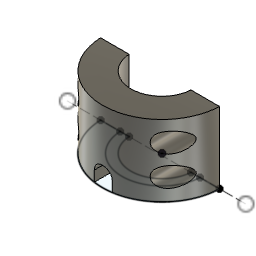
sphere_PS3 v1 (Autodesk Fusion 360 design; units mm, degrees)
Autodesk Fusion 360 part; units mm, degrees
sketch "Skizze1" plane through (0, 0, 0) normal (0, 0, 1) x (1, 0, 0)
  line L0 (-46.6781, -1) -> (43.3215, -1) construction
  arc A0 (-29.9833, -1) -> (29.9833, -1) centre (0, 0) ccw
  arc A1 (-20.1252, -1) -> (20.1252, -1) centre (0, 0) ccw
  arc A2 (-15.618, -1) -> (15.618, -1) centre (0, 0) ccw
  line L1 (15.618, -1) -> (29.9833, -1)
  line L2 (-15.618, -1) -> (-29.9833, -1)
  point P0 (-29.9833, -1)
  point P1 (-20.1252, -1)
  point P2 (-15.618, -1)
  point P3 (15.618, -1)
  point P4 (20.1252, -1)
  point P5 (29.9833, -1)
  dimension "d6" = 1
  dimension "d7" = 30
  dimension "d8" = 20.15
  dimension "d9" = 15.65
  constraint horizontal L0
  constraint coincident L0 P0
  constraint coincident L0 P1
  constraint coincident L0 P2
  constraint coincident L0 P3
  constraint coincident L0 P4
  constraint coincident L0 P5
  constraint coincident P5 A0.end
  constraint coincident P0 A0.start
  constraint coincident A0.centre A1.centre
  constraint coincident P4 A1.end
  constraint coincident P1 A1.start
  constraint coincident P3 A2.end
  constraint coincident P2 A2.start
  measures "d6" distance of A0.centre L0
  measures "d7" radius of A0
  measures "d8" radius of A1
  measures "d9" radius of A2
extrude "Extrusion1" add sketch "Skizze1" along normal blind 36
extrude "Extrusion2" cut sketch "Skizze1" along normal blind 5.3 contours A1 A2 L1 L2
sketch "Skizze3" plane through (0, -1, 0) normal (0, 1, 0) x (-1, 0, 0)
  line L0 (20.1252, 5.3) -> (20.1252, 0)
  line L1 (20.1252, 0) -> (29.9833, 0)
  line L2 (29.9833, 0) -> (29.9833, 36)
  line L3 (29.9833, 36) -> (15.618, 36)
  line L4 (15.618, 36) -> (15.618, 5.3)
  line L5 (15.618, 5.3) -> (20.1252, 5.3)
  line L6 (-23, 38.9334) -> (-23, -25) construction
  line L7 (23, 38.9334) -> (23, -33.2487) construction
  line L8 (-52.1355, 10.8) -> (51.6739, 10.8) construction
  line L9 (-50.0712, 25.8) -> (44.4743, 25.8) construction
  circle A0 centre (-23, 25.8) radius 1.75
  circle A1 centre (-23, 10.8) radius 1.75
  circle A2 centre (23, 25.8) radius 1.75
  circle A3 centre (23, 10.8) radius 1.75
  line L10 (-51.02, 5.3) -> (55, 5.3) construction
  line L11 (0, 38.1175) -> (0, -20) construction
  line L12 (-4.5, 5.3) -> (4.5, 5.3)
  line L13 (4.5, 5.3) -> (4.5, -4.7)
  line L14 (4.5, -4.7) -> (-4.5, -4.7)
  line L15 (-4.5, -4.7) -> (-4.5, 5.3)
  arc A4 (4.5, 5.3) -> (-4.5, 5.3) centre (0, 5.3) ccw
  point P0 (-23, 25.8)
  point P1 (-23, 10.8)
  point P2 (23, 25.8)
  point P3 (23, 10.8)
  dimension "d14" = 10.8
  dimension "d15" = 25.8
  dimension "d17" = 3.5
  dimension "d18" = 3.5
  dimension "d19" = 3.5
  dimension "d20" = 3.5
  dimension "d21" = 5.3
  dimension "d29" = 23
  dimension "d30" = 23
  constraint vertical L6
  constraint perpendicular L3 L7
  constraint horizontal L8
  constraint perpendicular L2 L9
  constraint coincident L9 P0
  constraint coincident L6 P0
  constraint coincident L6 P1
  constraint coincident L8 P1
  constraint coincident L9 P2
  constraint coincident L7 P2
  constraint coincident L7 P3
  constraint coincident L8 P3
  constraint coincident P0 A0.centre
  constraint coincident P1 A1.centre
  constraint coincident P2 A2.centre
  constraint coincident P3 A3.centre
  constraint horizontal L10
  constraint vertical L11
  constraint coincident origin L11
  constraint horizontal L12
  constraint vertical L13
  constraint horizontal L14
  constraint vertical L15
  constraint midpoint L12 A4.centre
  measures "d14" distance of L8 origin
  measures "d15" distance of origin L9
  measures "d17" diameter of A3
  measures "d18" diameter of A2
  measures "d19" diameter of A0
  measures "d20" diameter of A1
  measures "d21" distance of origin L10
  measures "d29" distance of L6 L11
  measures "d30" distance of L7 L11
extrude "Extrusion3" cut sketch "Skizze3" against normal blind 100 contours A0 | A1 | A2 | A3 | L12 A4 | L12 L13 L14 L15
ref_plane "Arbeitsebene1" through (0, -30, 0) normal (0, 1, 0) x (0, 0, 1)
sketch "Skizze5" plane through (0, -30, 0) normal (0, 1, 0) x (1, 0, 0)
  line L0 (23, -32.4719) -> (23, 19) construction
  line L1 (-23, -30.4738) -> (-23, 19) construction
  line L2 (48, -10.8) -> (-39, -10.8) construction
  line L3 (47, -25.8) -> (-45, -25.8) construction
  circle A0 centre (23, -25.8) radius 5
  circle A1 centre (23, -10.8) radius 5
  circle A2 centre (-23, -25.8) radius 5
  circle A3 centre (-23, -10.8) radius 5
  dimension "d27" = 23
  dimension "d31" = 23
  dimension "d32" = 10.8
  dimension "d33" = 25.8
  dimension "d34" = 10
  dimension "d35" = 10
  dimension "d36" = 10
  dimension "d37" = 10
  constraint vertical L0
  constraint vertical L1
  constraint perpendicular L1 L2
  constraint perpendicular L0 L3
  constraint coincident L0 A0.centre
  constraint coincident L3 A0.centre
  constraint coincident L2 A1.centre
  constraint coincident L0 A1.centre
  constraint coincident L1 A2.centre
  constraint coincident L3 A2.centre
  constraint coincident L2 A3.centre
  constraint coincident L1 A3.centre
  measures "d27" distance of L1 origin
  measures "d31" distance of L0 origin
  measures "d32" distance of origin L2
  measures "d33" distance of L3 origin
  measures "d34" diameter of A2
  measures "d35" diameter of A3
  measures "d36" diameter of A0
  measures "d37" diameter of A1
extrude "Extrusion4" cut sketch "Skizze5" along normal blind 26
